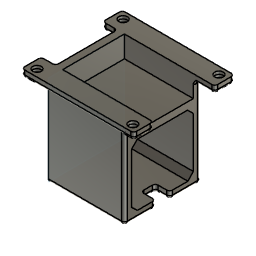
_motor bracket.44d059b8-f0a0-49a9-bc9c-bc6a08ed9233 (Autodesk Fusion 360 design; units mm, degrees)
Autodesk Fusion 360 part; units mm, degrees
sketch "Sketch1" plane through (0, 0, 0) normal (0, 0, 1) x (1, 0, 0)
  line L0 (0, 0) -> (48, 0)
  line L1 (48, 0) -> (48, 53)
  line L2 (48, 53) -> (0, 53)
  line L3 (0, 53) -> (0, 0)
  dimension "d1" = 48
  dimension "d2" = 53
  constraint horizontal L0
  constraint vertical L1
  constraint horizontal L2
  constraint vertical L3
  constraint coincident L0.start L3.end
  measures "d1" distance of L0.start L0.end
  measures "d2" distance of L0.start L2.end
extrude "Extrude1" add sketch "Sketch1" along normal blind 5
sketch "Sketch2" plane through (0, 0, 5) normal (0, 0, 1) x (-1, 0, 0)
  line L0 (0, -53) -> (0, 0)
  line L1 (0, 0) -> (-48, 0)
  line L2 (-48, 0) -> (-48, -53)
  line L3 (-48, -53) -> (0, -53)
  line L4 (0, 0) -> (-48, 0)
  line L5 (-48, 0) -> (-48, -5)
  line L6 (-48, -5) -> (0, -5)
  line L7 (0, -5) -> (0, 0)
  line L8 (0, -53) -> (-48, -53)
  line L9 (-48, -53) -> (-48, -48)
  line L10 (-48, -48) -> (0, -48)
  line L11 (0, -48) -> (0, -53)
  dimension "d5" = 48
  dimension "d6" = 5
  dimension "d7" = 48
  dimension "d8" = 5
  constraint horizontal L4
  constraint vertical L5
  constraint horizontal L6
  constraint vertical L7
  constraint coincident L0.end L1.start
  constraint horizontal L8
  constraint vertical L9
  constraint horizontal L10
  constraint vertical L11
  constraint coincident L0.start L3.end
  measures "d5" distance of L0.end L1.end
  measures "d6" distance of L0.end L6.end
  measures "d7" distance of L0.start L2.end
  measures "d8" distance of L0.start L10.end
extrude "Extrude2" add sketch "Sketch2" along normal blind 58 contours L0 L2 L3 L8 L9 L10 L11 | L0 L1 L2 L4 L5 L6 L7
sketch "Sketch3" plane through (48, 0, 0) normal (1, 0, 0) x (0, 1, 0)
  line L0 (0, 0) -> (53, 0)
  line L1 (53, 0) -> (53, 63)
  line L2 (53, 63) -> (48, 63)
  line L3 (48, 63) -> (48, 5)
  line L4 (48, 5) -> (5, 5)
  line L5 (5, 5) -> (5, 63)
  line L6 (5, 63) -> (0, 63)
  line L7 (0, 63) -> (0, 0)
  line L8 (11, 0) -> (42, 0)
  line L9 (42, 0) -> (42, 10)
  line L10 (42, 10) -> (11, 10)
  line L11 (11, 10) -> (11, 0)
  line L12 (42, 0) -> (11, 10) construction
  line L13 (31.5, 0) -> (21.5, 0)
  line L14 (21.5, 0) -> (21.5, 10)
  line L15 (21.5, 10) -> (31.5, 10)
  line L16 (31.5, 10) -> (31.5, 0)
  line L17 (31.5, 0) -> (21.5, 10) construction
  line L18 (21.5, 0) -> (31.5, 10) construction
  line L19 (9, 5) -> (5, 8.7583)
  line L20 (5, 8.7583) -> (1.4689, 5)
  line L21 (1.4689, 5) -> (5.4689, 1.2417)
  line L22 (5.4689, 1.2417) -> (9, 5)
  line L23 (44.2408, 5) -> (48, 9)
  line L24 (48, 9) -> (51.759, 5.4674)
  line L25 (51.759, 5.4674) -> (47.9998, 1.4674)
  line L26 (47.9998, 1.4674) -> (44.2408, 5)
  point P0 (26.5, 5)
  point P1 (26.5, 5)
  dimension "d11" = 31
  dimension "d12" = 10
  dimension "d36" = 10
  dimension "d37" = 10
  constraint horizontal L8
  constraint perpendicular L8 L9
  constraint parallel L8 L10
  constraint parallel L9 L11
  constraint coincident L12 P1
  constraint midpoint L4 P1
  constraint horizontal L13
  constraint perpendicular L13 L14
  constraint parallel L13 L15
  constraint parallel L14 L16
  constraint coincident L17 P1
  constraint coincident L18 P1
  constraint coincident P1 P0
  constraint perpendicular L19 L20
  constraint parallel L19 L21
  constraint parallel L20 L22
  constraint coincident L5 L19.end
  constraint coincident L4 L19.start
  constraint perpendicular L23 L24
  constraint parallel L23 L25
  constraint parallel L24 L26
  constraint coincident L3 L23.end
  constraint coincident L4 L23.start
  measures "d11" distance of L9.end L10.end
  measures "d12" distance of L8.end L9.end
  measures "d36" distance of L14.end L15.end
  measures "d37" distance of L13.end L14.end
extrude "Extrude3" add sketch "Sketch3" against normal blind 48 contours L4 L5 L19 | L3 L4 L23
extrude "Extrude8" cut sketch "Sketch3" against normal blind 10 contours L0 L4 L8 L13 L14 L16
sketch "Sketch10" plane through (0, 0, 63) normal (0, 0, 1) x (-1, 0, 0)
  line L0 (0, -5) -> (0, 0)
  line L1 (0, 0) -> (-48, 0)
  line L2 (-48, 0) -> (-48, -5)
  line L3 (-48, -5) -> (0, -5)
  line L4 (0, 0) -> (-24, 0)
  line L5 (-24, 0) -> (-24, -26.5)
  line L6 (-24, -26.5) -> (0, -26.5)
  line L7 (0, -26.5) -> (0, 0)
  line L8 (-63, 8.5) -> (15, 8.5)
  line L9 (15, 8.5) -> (15, -61.5)
  line L10 (15, -61.5) -> (-63, -61.5)
  line L11 (-63, -61.5) -> (-63, 8.5)
  line L12 (-63, 8.5) -> (15, -61.5) construction
  line L13 (15, 8.5) -> (-63, -61.5) construction
  line L14 (25.7546, 3.5) -> (-73.7546, 3.5)
  line L15 (-73.7546, 3.5) -> (-73.7546, -56.5)
  line L16 (-73.7546, -56.5) -> (25.7546, -56.5)
  line L17 (25.7546, -56.5) -> (25.7546, 3.5)
  line L18 (25.7546, 3.5) -> (-73.7546, -56.5) construction
  line L19 (-73.7546, 3.5) -> (25.7546, -56.5) construction
  circle A0 centre (-57.4286, -56.5) radius 3
  circle A1 centre (9.4286, -56.5) radius 3
  circle A2 centre (9.4286, 3.5) radius 3
  circle A3 centre (-57.4286, 3.5) radius 3
  point P0 (-24, -26.5)
  point P1 (-24, -26.5)
  dimension "d48" = 24
  dimension "d49" = 26.5
  dimension "d50" = 78
  dimension "d51" = 70
  dimension "d78" = 60
  dimension "d79" = 6
  dimension "d80" = 6
  dimension "d81" = 6
  dimension "d82" = 6
  constraint horizontal L4
  constraint vertical L5
  constraint horizontal L6
  constraint vertical L7
  constraint coincident L0.end L1.start
  constraint horizontal L8
  constraint perpendicular L8 L9
  constraint parallel L8 L10
  constraint parallel L9 L11
  constraint coincident L12 P1
  constraint coincident L13 P1
  constraint coincident P1 P0
  constraint horizontal L14
  constraint perpendicular L14 L15
  constraint parallel L14 L16
  constraint parallel L15 L17
  constraint coincident L18 P1
  constraint coincident L19 P1
  constraint coincident L16 A0.centre
  constraint coincident L13 A0.centre
  constraint coincident L12 A1.centre
  constraint coincident L16 A1.centre
  constraint coincident L14 A2.centre
  constraint coincident L13 A2.centre
  constraint coincident L14 A3.centre
  constraint coincident L12 A3.centre
  measures "d48" distance of L0.end L4.end
  measures "d49" distance of L0.end L6.end
  measures "d50" distance of L9.end L10.end
  measures "d51" distance of L8.end L9.end
  measures "d78" distance of L14.end L15.end
  measures "d79" diameter of A0
  measures "d80" diameter of A1
  measures "d81" diameter of A2
  measures "d82" diameter of A3
extrude "Extrude10" add sketch "Sketch10" along normal blind 5 contours L0 L1 L3 L4 L5 L7 | L3 L5 L6 L7 | L1 L2 L3 L5 | L8 L9 L11 L14 A2 A3 | L9 L11 L14 L16 A0 A1 A2 A3 | L9 L10 L11 L16 A0 A1 | L14 A3 | L14 A3 | L14 A2 | L14 A2 | L16 A0 | L16 A0 | L16 A1 | L16 A1
sketch "Sketch14" plane through (0, 0, 68) normal (0, 0, 1) x (-1, 0, 0)
  line L0 (-63, -61.5) -> (15, -61.5)
  line L1 (15, -61.5) -> (15, 8.5)
  line L2 (15, 8.5) -> (-63, 8.5)
  line L3 (-63, 8.5) -> (-63, -61.5)
  line L4 (15, -5) -> (-85, -5)
  line L5 (-85, -5) -> (-85, -48)
  line L6 (-85, -48) -> (15, -48)
  line L7 (15, -48) -> (15, -5)
  dimension "d58" = 100
  dimension "d59" = 43
  constraint horizontal L4
  constraint vertical L5
  constraint horizontal L6
  constraint vertical L7
  constraint coincident L1 L4.start
  measures "d58" distance of L4.start L4.end
  measures "d59" distance of L4.start L6.end
extrude "Extrude12" cut sketch "Sketch14" against normal blind 5 contours L1 L3 L4 L6 L7
extrude "Extrude17" cut sketch "Sketch10" along normal blind 5 contours L14 A3 | L14 A3 | L14 A2 | L14 A2 | L16 A0 | L16 A0 | L16 A1 | L16 A1
sketch "Sketch22" plane through (0, 0, 63) normal (0, 0, -1) x (1, 0, 0)
  circle A0 centre (-9.4286, 3.5) radius 3
  circle A1 centre (57.4286, 3.5) radius 3
  line L0 (48, -5) -> (63, -5)
  line L1 (63, -5) -> (63, 8.5)
  line L2 (63, 8.5) -> (-15, 8.5)
  line L3 (-15, 8.5) -> (-15, -5)
  line L4 (-15, -5) -> (0, -5)
  line L5 (0, -5) -> (0, 0)
  line L6 (0, 0) -> (48, 0)
  line L7 (48, 0) -> (48, -5)
  circle A2 centre (-9.4286, 3.5) radius 4.5
  circle A3 centre (57.4286, 3.5) radius 4.5
  dimension "d85" = 9
  dimension "d86" = 9
  constraint concentric A0 A2
  constraint concentric A1 A3
  measures "d85" diameter of A2
  measures "d86" diameter of A3
extrude "Extrude18" cut sketch "Sketch22" against normal blind 3 contours A2 | A3
sketch "Sketch23" plane through (0, 0, 63) normal (0, 0, -1) x (1, 0, 0)
  circle A0 centre (-9.4286, -56.5) radius 3
  circle A1 centre (57.4286, -56.5) radius 3
  line L0 (63, -48) -> (48, -48)
  line L1 (48, -48) -> (48, -53)
  line L2 (48, -53) -> (0, -53)
  line L3 (0, -53) -> (0, -48)
  line L4 (0, -48) -> (-15, -48)
  line L5 (-15, -48) -> (-15, -61.5)
  line L6 (-15, -61.5) -> (63, -61.5)
  line L7 (63, -61.5) -> (63, -48)
  circle A2 centre (-9.4286, -56.5) radius 4.5
  circle A3 centre (57.4286, -56.5) radius 4.5
  dimension "d89" = 9
  dimension "d90" = 9
  constraint concentric A0 A2
  constraint concentric A1 A3
  measures "d89" diameter of A2
  measures "d90" diameter of A3
extrude "Extrude19" cut sketch "Sketch23" against normal blind 3 contours A2 | A3
extrude "Extrude20" add 1 faces at (0, 51.3333, 24) along direction (-1, 0, 0) blind 5
sketch "Sketch24" plane through (0, 48, 0) normal (0, -1, 0) x (1, 0, 0)
  line L0 (-5, 9) -> (48, 9)
  line L1 (48, 9) -> (48, 63)
  line L2 (48, 63) -> (63, 63)
  line L3 (63, 63) -> (63, 68)
  line L4 (63, 68) -> (-15, 68)
  line L5 (-15, 68) -> (-15, 63)
  line L6 (-15, 63) -> (-5, 63)
  line L7 (-5, 63) -> (-5, 9)
  line L8 (-5, 63) -> (0, 63)
  line L9 (0, 63) -> (0, 0)
  line L10 (0, 0) -> (-5, 0)
  line L11 (-5, 0) -> (-5, 63)
  constraint horizontal L8
  constraint vertical L9
  constraint horizontal L10
  constraint vertical L11
  constraint coincident L9.end L10.start
  constraint coincident L6.end L7.start
extrude "Extrude21" add sketch "Sketch24" along normal blind 45 contours L0 L7 L8 L9 L11 | L0 L9 L10 L11
sketch "Sketch25" plane through (-5, 0, 0) normal (-1, 0, 0) x (0, -1, 0)
  line L0 (-48, 63) -> (-53, 63)
  line L1 (-53, 63) -> (-53, 0)
  line L2 (-53, 0) -> (0, 0)
  line L3 (0, 0) -> (0, 63)
  line L4 (0, 63) -> (-5, 63)
  line L5 (-5, 63) -> (-48, 63)
extrude "Extrude22" add 1 faces at (-3.3333, 33.6667, 63) along direction (0, 0, 1) blind 5
sketch "Sketch26" plane through (-5, 0, 0) normal (-1, 0, 0) x (0, -1, 0)
  line L0 (0, 0) -> (-26.5, 0)
  line L1 (-26.5, 0) -> (-26.5, 25.5)
  line L2 (-26.5, 25.5) -> (0, 25.5)
  line L3 (0, 25.5) -> (0, 0)
  circle A0 centre (-26.5, 25.5) radius 12.5
  dimension "d101" = 26.5
  dimension "d102" = 25.5
  dimension "d103" = 25
  constraint horizontal L0
  constraint vertical L1
  constraint horizontal L2
  constraint vertical L3
  constraint coincident L0.start L3.end
  constraint coincident L1.end L2.start
  measures "d101" distance of L0.start L0.end
  measures "d102" distance of L0.start L2.end
  measures "d103" diameter of A0
extrude "Extrude23" cut sketch "Sketch26" against normal blind 5 contours L1 L2 A0 | L1 L2 A0
sketch "Sketch27" plane through (-5, 0, 0) normal (-1, 0, 0) x (0, -1, 0)
  line L0 (0, 0) -> (-26.5, 0)
  line L1 (-26.5, 0) -> (-26.5, 25.5)
  line L2 (-26.5, 25.5) -> (0, 25.5)
  line L3 (0, 25.5) -> (0, 0)
  line L4 (-41.5, 10.5) -> (-11.5, 10.5)
  line L5 (-11.5, 10.5) -> (-11.5, 40.5)
  line L6 (-11.5, 40.5) -> (-41.5, 40.5)
  line L7 (-41.5, 40.5) -> (-41.5, 10.5)
  line L8 (-41.5, 10.5) -> (-11.5, 40.5) construction
  line L9 (-11.5, 10.5) -> (-41.5, 40.5) construction
  circle A0 centre (-11.5, 10.5) radius 1.5
  circle A1 centre (-41.5, 10.5) radius 1.5
  circle A2 centre (-11.5, 40.5) radius 1.5
  circle A3 centre (-41.5, 40.5) radius 1.5
  point P0 (-26.5, 25.5)
  dimension "d106" = 26.5
  dimension "d107" = 25.5
  dimension "d108" = 30
  dimension "d109" = 30
  dimension "d110" = 3
  dimension "d111" = 3
  dimension "d112" = 3
  dimension "d113" = 3
  constraint horizontal L0
  constraint vertical L1
  constraint horizontal L2
  constraint vertical L3
  constraint coincident L0.start L3.end
  constraint horizontal L4
  constraint perpendicular L4 L5
  constraint parallel L4 L6
  constraint parallel L5 L7
  constraint coincident L8 P0
  constraint coincident L9 P0
  constraint coincident P0 L1.end
  constraint coincident L4.end L5.start
  constraint coincident L4.start L7.end
  constraint coincident L5.end L6.start
  constraint coincident L6.end L7.start
  measures "d106" distance of L0.start L0.end
  measures "d107" distance of L0.start L2.end
  measures "d108" distance of L5.end L6.end
  measures "d109" distance of L4.end L5.end
  measures "d110" diameter of A0
  measures "d111" diameter of A1
  measures "d112" diameter of A2
  measures "d113" diameter of A3
extrude "Extrude24" cut sketch "Sketch27" against normal blind 5 contours L4 L7 A1 | L4 L7 A1 | L4 L5 A0 | L4 L5 A0 | L5 L6 A2 | L5 L6 A2 | L6 L7 A3 | L6 L7 A3
fillet "Fillet2" radius 2 38 edges at (63, 61.5, 65.5) (24, 61.5, 63) (63, 54.75, 63) (55.5, 48, 63) (48, 53, 31.5) (48, 42.25, 0) (38, 26.5, 0) (43, 21.5, 0) (38, 21.5, 2.5) (38, 31.5, 2.5) (43, 31.5, 0) (48, 10.75, 0) (21.5, 0, 0) (21.5, 53, 0) (55.5, 5, 63) (48, 50.5, 63) (48, 2.5, 63) (48, 0, 31.5) (63, 48, 65.5) (63, 5, 65.5) (63, -8.5, 65.5) (63, -1.75, 63) (24, -8.5, 63) (21.5, 0, 63) (-15, -8.5, 65.5) (-15, -1.75, 63) (-10, 5, 63) (-5, 48, 65.5) (-10, 48, 63) (-15, 48, 65.5) (-15, 54.75, 63) (-15, 61.5, 65.5) (-5, 5, 65.5) (-5, 38.1541, 30.0202) (-15, 5, 65.5) (21.5, 53, 63) (48, 21.5, 2.5) (48, 31.5, 2.5)
sketch "Sketch29" plane through (0, 5, 0) normal (0, 1, 0) x (-1, 0, 0)
  line L0 (-48, 61.5359) -> (-48, 8.7583)
  line L1 (-48, 8.7583) -> (0, 8.7583)
  line L2 (0, 8.7583) -> (0, 68)
  line L3 (0, 68) -> (-61, 68)
  line L4 (-61, 68) -> (-61, 65)
  line L5 (-61, 65) -> (-50, 65)
  spline S0 degree 3 poles (-48, 61.5359) (-48, 61.7908) (-48.0389, 62.0661) (-48.1892, 62.5981) (-48.2999, 62.855) (-48.6065, 63.4245) (-48.8579, 63.7703) (-49.4173, 64.4184) (-49.7229, 64.7229) (-50, 65) knots 1.011064 1.011064 1.011064 1.011064 1.087528 1.087528 1.163991 1.163991 1.281554 1.281554 1.399117 1.399117 1.399117 1.399117
  line L6 (0, 8.7583) -> (-48, 8.7583)
  line L7 (-48, 8.7583) -> (-48, 53)
  line L8 (-48, 53) -> (0, 53)
  line L9 (0, 53) -> (0, 8.7583)
  line L10 (-48, 53) -> (0, 53)
  line L11 (0, 53) -> (0, 48)
  line L12 (0, 48) -> (-48, 48)
  line L13 (-48, 48) -> (-48, 53)
  dimension "d118" = 48
  dimension "d119" = 48
  dimension "d120" = 5
  constraint horizontal L6
  constraint vertical L7
  constraint horizontal L8
  constraint vertical L9
  constraint coincident L1.end L2.start
  constraint horizontal L10
  constraint vertical L11
  constraint horizontal L12
  constraint vertical L13
  measures "d118" distance of L1.end L0.end
  measures "d119" distance of L7.end L8.end
  measures "d120" distance of L7.end L12.end
extrude "Extrude25" add sketch "Sketch29" along normal blind 45 contours L0 L2 L7 L8 L9 L10 L11 L12 L13
chamfer "Chamfer1" distance 4 angle 45 2 edges at (24, 5, 48) (24, 48, 48)
